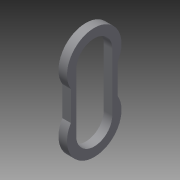
# Autodesk Inventor part: Sensor support
Saved by Autodesk Inventor 2015 (Build 190159000, 159)
## iProperties
Created: 2016-06-05
Part Number: Sensor support
Material: Generic
Document SubType Name: Modeling
Designer: EriveltonDell
Density: 1 g/cm^3
Appearance: Default
Author: EriveltonDell
Autodesk Inventor part; units mm, degrees
ref_plane "YZ Plane" through (0, 0, 0) normal (1, 0, 0) x (0, 1, 0)
ref_plane "XZ Plane" through (0, 0, 0) normal (0, 1, 0) x (-1, 0, 0)
ref_plane "XY Plane" through (0, 0, 0) normal (0, 0, 1) x (1, 0, 0)
sketch "Sketch1" plane through (0, 0, 0) normal (1, 0, 0) x (0, 1, 0)
  arc A0 (18.5, 35) -> (1.5, 35) centre (10, 35) ccw
  arc A1 (1.5, 8) -> (18.5, 8) centre (10, 8) ccw
  arc A2 (21, 28.4426) -> (-1, 28.4426) centre (10, 35) ccw
  line L0 (18.5, 8) -> (18.5, 35)
  line L1 (1.5, 35) -> (1.5, 8)
  line L2 (21, 28.4426) -> (21, 14.5574)
  line L3 (-1, 14.5574) -> (-1, 28.4426)
  arc A3 (-1, 14.5574) -> (21, 14.5574) centre (10, 8) ccw
  dimension "d12" = 17
  dimension "d13" = 17
  constraints: 8 end point, 8 point on circle, 4 centre point, 2 coincident, 1 parallel
  measures "d12" diameter of A0
  measures "d13" diameter of A1
extrude "Extrusion1" add sketch "Sketch1" along normal blind 4
body "Solid1"
